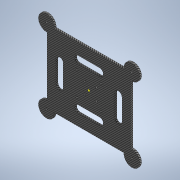
# Autodesk Inventor part: Payload bay KPM
Saved by Autodesk Inventor 2020.3 (Build 243373000, 373)
## iProperties
Created: 2020-10-15
Part Number: Payload bay KPM
Material: CFRP
Document SubType Name: Modeling
Designer: Krishna Makhija
Density: 1.43 g/cm^3
Appearance: Carbon Fiber
Author: Krishna Makhija
Autodesk Inventor part; units mm, degrees
ref_plane "YZ Plane" through (0, 0, 0) normal (1, 0, 0) x (0, 1, 0)
ref_plane "XZ Plane" through (0, 0, 0) normal (0, 1, 0) x (-1, 0, 0)
ref_plane "XY Plane" through (0, 0, 0) normal (0, 0, 1) x (1, 0, 0)
sketch "Sketch1" plane through (0, 0, 0) normal (0, 0, 1) x (1, 0, 0)
  point P0 (0, 0)
sketch "Sketch2" plane through (0, 0, 0) normal (0, 0, 1) x (1, 0, 0)
  line L0 (78.4999, -68.5) -> (-78.4999, -68.5)
  line L1 (-78.4999, -68.5) -> (-78.4999, 68.5)
  line L2 (-78.4999, 68.5) -> (78.4999, 68.5)
  line L3 (78.4999, 68.5) -> (78.4999, -68.5)
  circle A0 centre (80, 70) radius 14.9999
  circle A1 centre (-80, 70) radius 14.9999
  circle A2 centre (-80, -70) radius 14.9999
  circle A3 centre (80, -70) radius 14.9999
  point P0 (78.4999, -55.0753)
  point P1 (78.4999, 55.0753)
  point P2 (65.0752, 68.5)
  point P3 (-65.0752, 68.5)
  point P4 (-78.4999, 55.0753)
  point P5 (-78.4999, -55.0753)
  point P6 (-65.0752, -68.5)
  point P7 (65.0752, -68.5)
  constraints: 8 end point, 4 centre point, 2 parallel, 1 horizontal, 1 perpendicular
extrude "Extrusion1" add sketch "Sketch2" along normal blind 3
sketch "Sketch5" plane through (0, 0, 3) normal (0, 0, 1) x (1, 0, 0)
  circle A0 centre (80, 70) radius 1.4999
  circle A1 centre (-80, 70) radius 1.4999
  circle A2 centre (-80, -70) radius 1.4999
  circle A3 centre (80, -70) radius 1.4999
  constraints: 4 centre point
extrude "Extrusion2" cut sketch "Sketch5" against normal blind 10
sketch "Sketch6" plane through (0, 0, 3) normal (0, 0, 1) x (1, 0, 0)
  point P0 (0, 0)
sketch "Cable cutouts" plane through (0, 0, 3) normal (0, 0, 1) x (1, 0, 0)
  line L0 (65.0752, 68.5) -> (-65.0752, 68.5) projected
  line L1 (-20.0003, 40) -> (20.0003, 40) construction
  line L2 (-20.0003, 33.4981) -> (20.0003, 33.4981)
  line L3 (20.0003, 46.5019) -> (-20.0003, 46.5019)
  arc A0 (-20.0003, 46.5019) -> (-20.0003, 33.4981) centre (-20.0003, 40) ccw
  arc A1 (20.0003, 33.4981) -> (20.0003, 46.5019) centre (20.0003, 40) ccw
  line L4 (-20.0003, -40) -> (20.0003, -40) construction
  line L5 (-20.0003, -46.5019) -> (20.0003, -46.5019)
  line L6 (20.0003, -33.4981) -> (-20.0003, -33.4981)
  arc A2 (-20.0003, -33.4981) -> (-20.0003, -46.5019) centre (-20.0003, -40) ccw
  arc A3 (20.0003, -46.5019) -> (20.0003, -33.4981) centre (20.0003, -40) ccw
  line L7 (55, -20.0003) -> (55, 20.0003) construction
  arc A4 (48.4981, -20.0003) -> (61.5019, -20.0003) centre (55, -20.0003) ccw
  arc A5 (61.5019, 20.0003) -> (48.4981, 20.0003) centre (55, 20.0003) ccw
  line L8 (48.4981, 20.0003) -> (48.4981, -20.0003)
  line L9 (61.5019, -20.0003) -> (61.5019, 20.0003)
  line L10 (-55, -20.0003) -> (-55, 20.0003) construction
  arc A6 (-61.5019, -20.0003) -> (-48.4981, -20.0003) centre (-55, -20.0003) ccw
  arc A7 (-48.4981, 20.0003) -> (-61.5019, 20.0003) centre (-55, 20.0003) ccw
  line L11 (-61.5019, 20.0003) -> (-61.5019, -20.0003)
  line L12 (-48.4981, -20.0003) -> (-48.4981, 20.0003)
  constraints: 32 end point, 16 point on circle, 16 tangent, 8 centre point, 4 parallel
extrude "Extrusion4" cut sketch "Cable cutouts" against normal blind 10
sketch "Pixhawk 3 Pro mount holes" plane through (0, 0, 3) normal (0, 0, 1) x (1, 0, 0)
  circle A0 centre (13.75, 10.75) radius 1.2498
  circle A1 centre (-7.75, 10.75) radius 1.2498
  circle A2 centre (-7.75, -10.75) radius 1.2498
  circle A3 centre (13.75, -10.75) radius 1.2498
  constraints: 4 centre point
extrude "Extrusion5" cut sketch "Pixhawk 3 Pro mount holes" against normal blind 10
sketch "Anti-vibration mount holes" plane through (0, 0, 3) normal (0, 0, 1) x (1, 0, 0)
  circle A0 centre (22.5, 22.5) radius 1.4999
  circle A1 centre (-22.5, 22.5) radius 1.4999
  circle A2 centre (-22.5, -22.5) radius 1.4999
  circle A3 centre (22.5, -22.5) radius 1.4999
  constraints: 4 centre point
extrude "Extrusion7" cut sketch "Anti-vibration mount holes" against normal blind 10
body "Solid1"
